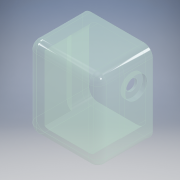
# Autodesk Inventor part: Case_Top
Saved by Autodesk Inventor 2020 (Build 240168000, 168)
## iProperties
Created: 2020-02-24
Part Number: Case_Top
Material: 일반
Document SubType Name: Modeling
Designer: Knowblesse
Density: 1 g/cm^3
Appearance: 기본값
Author: Knowblesse
## iProperties of the stored document _3D 인쇄.ipt
Created: 2020-02-24
Part Number: _3D 인쇄
Material: 일반
Document SubType Name: Modeling
Designer: Knowblesse
Density: 1 g/cm^3
Appearance: 기본값
Author: Knowblesse
Autodesk Inventor part; units mm, degrees
ref_plane "YZ Plane" through (0, 0, 0) normal (1, 0, 0) x (0, 1, 0)
ref_plane "XZ Plane" through (0, 0, 0) normal (0, 1, 0) x (-1, 0, 0)
ref_plane "XY Plane" through (0, 0, 0) normal (0, 0, 1) x (1, 0, 0)
sketch "스케치1" plane through (0, 0, 0) normal (0, 0, 1) x (1, 0, 0)
  line L0 (0, 0) -> (13, 0)
  line L1 (13, 0) -> (13, 15.5)
  line L2 (13, 15.5) -> (0, 15.5)
  line L3 (0, 15.5) -> (0, 0)
  line L4 (-1.5, 17) -> (14.5, 17)
  line L5 (14.5, 17) -> (14.5, -1.5)
  line L6 (14.5, -1.5) -> (-1.5, -1.5)
  line L7 (-1.5, -1.5) -> (-1.5, 17)
  dimension "d0" = 13
  dimension "d1" = 15.5
  dimension "d2" = 1.5
  constraints: 16 end point, 4 parallel, 2 perpendicular, 1 horizontal, 3 other
  measures "d0" distance of L1.end L2.end
  measures "d1" distance between parallel lines of L0 L2
  measures "d2" distance between parallel lines of L2 L4
extrude "돌출1" add sketch "스케치1" along normal blind 5
sketch "스케치2" plane through (0, 0, 5) normal (0, 0, 1) x (1, 0, 0)
  line L0 (-1.5, 17) -> (-1.5, -1.5) projected
  line L1 (-1.5, -1.5) -> (14.5, -1.5) projected
  line L2 (14.5, -1.5) -> (14.5, 17) projected
  line L3 (14.5, 17) -> (-1.5, 17) projected
  line L4 (13, 0) -> (0, 0) projected
  line L5 (0, 0) -> (0, 15.5) projected
  line L6 (0, 15.5) -> (13, 15.5) projected
  line L7 (13, 15.5) -> (13, 0) projected
  line L8 (1, 15.5) -> (1, 0)
  line L9 (13, 0) -> (0, 0) projected
  line L10 (12, 15.5) -> (12, 0)
  line L11 (0, 15.5) -> (13, 15.5) projected
  point P0 (12, 15.5)
  dimension "d5" = 1
  dimension "d6" = 1
  constraints: 4 end point, 4 point on line, 2 perpendicular
  measures "d5" distance between parallel lines of L5 L8
  measures "d6" distance between parallel lines of L7 L10
extrude "돌출2" add sketch "스케치2" along normal blind 6 contours L3 L2 L1 L0 | L4 L10 L6 L7 | L4 L5 L6 L8
fillet "모깎기1" radius 2 4 edges at (0, 15.5, 2.5) (13, 15.5, 2.5) (13, 0, 2.5) (0, 0, 2.5)
sketch "스케치3" plane through (0, 0, 11) normal (0, 0, 1) x (1, 0, 0)
  line L0 (-1.5, -1.5) -> (14.5, -1.5) projected
  line L1 (14.5, -1.5) -> (14.5, 17) projected
  line L2 (14.5, 17) -> (-1.5, 17) projected
  line L3 (-1.5, 17) -> (-1.5, -1.5) projected
  line L4 (11, 0) -> (2, 0) projected
  arc A0 (1, 0.2679) -> (2, 0) centre (2, 2) ccw projected
  line L5 (1, 0.2679) -> (1, 15.2321) projected
  arc A1 (2, 15.5) -> (1, 15.2321) centre (2, 13.5) ccw projected
  line L6 (2, 15.5) -> (11, 15.5) projected
  arc A2 (12, 15.2321) -> (11, 15.5) centre (11, 13.5) ccw projected
  line L7 (12, 15.2321) -> (12, 0.2679) projected
  arc A3 (11, 0) -> (12, 0.2679) centre (11, 2) ccw projected
  point P0 (0, 0)
extrude "돌출3" add sketch "스케치3" along normal blind 1.5 contours L3 L2 L1 L0 | L4 A0 L5 A1 L6 A2 L7 A3
sketch "스케치4" plane through (14.5, -1.5, 0) normal (1, 0, 0) x (0, 0, -1)
  line L0 (-5, 15) -> (-5, 3.5) projected
  line L1 (-11, 17) -> (0, 17) projected
  point P0 (0, 1.5)
  point P1 (-3.75, 12.5)
  dimension "d12" = 1.25
  dimension "d14" = 4.5
  measures "d12" distance from line of L0 point (-3.75, 12.5)
  measures "d14" distance from line of L1 point (-3.75, 12.5)
hole "구멍1" at (14.5, 11, 3.75) direction (-1, 0, 0) diameter 2.5 depth 1.5 tip angle 118 counterbore diameter 5 counterbore depth 1
fillet "모깎기2" radius 2 8 edges at (14.5, -1.5, 6.25) (-1.5, -1.5, 6.25) (14.5, 17, 6.25) (-1.5, 17, 6.25) (14.5, 7.75, 12.5) (6.5, -1.5, 12.5) (-1.5, 7.75, 12.5) (6.5, 17, 12.5)
